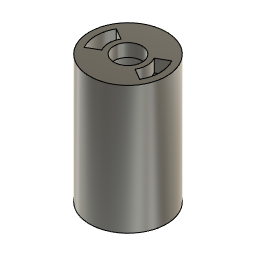
PDMSmould_holder (Autodesk Fusion 360 design; units mm, degrees)
Autodesk Fusion 360 part; units mm, degrees
sketch "Sketch1" plane through (0, 0, 0) normal (0, 0, 1) x (1, 0, 0)
  circle A0 centre (0, 0) radius 15
  dimension "d2" = 30
  constraint coincident A0.centre origin
  measures "d2" diameter of A0
extrude "Extrude1" add sketch "Sketch1" along normal blind 50
sketch "Sketch2" plane through (0, 0, 50) normal (0, 0, 1) x (-1, 0, 0)
  circle A0 centre (0, 0) radius 15
  circle A1 centre (0, 0) radius 12.5
  dimension "d5" = 25
  constraint concentric A0 A1
  measures "d5" diameter of A1
extrude "Extrude2" cut sketch "Sketch2" against normal blind 45 contours A1
sketch "Sketch4" plane through (0, 0, 50) normal (0, 0, 1) x (-1, 0, 0)
  circle A0 centre (0, 0) radius 12.5
  circle A1 centre (0, 0) radius 15
  circle A2 centre (0, 0) radius 15
  circle A3 centre (0, 0) radius 5.5
  dimension "d8" = 11
  constraint coincident A0.centre A1.centre
  measures "d8" diameter of A3
extrude "Extrude3" add sketch "Sketch4" against normal blind 5 contours A0
sketch "Sketch5" plane through (0, 0, 50) normal (0, 0, 1) x (-1, 0, 0)
  circle A0 centre (0, 0) radius 5.5
  circle A1 centre (0, 0) radius 15
  circle A2 centre (0, 0) radius 12.5
  circle A3 centre (0, 0) radius 7.5
  line L0 (0, 0) -> (12.5, 0) construction
  line L1 (0, 0) -> (-10.8253, 6.25)
  line L2 (0, 0) -> (12.5, 0) construction
  line L3 (0, 0) -> (-10.8253, -6.25)
  line L4 (0, 0) -> (12.5, 0) construction
  line L5 (0, 0) -> (10.8253, 6.25)
  line L6 (-10.8253, 6.25) -> (14.1746, 6.25) construction
  line L7 (0, 0) -> (10.8253, -6.25)
  line L8 (0, 0) -> (12.5, 0) construction
  dimension "d11" = 25
  dimension "d12" = 15
  dimension "d14" = 150
  dimension "d15" = 150
  dimension "d18" = 30
  constraint concentric A0 A2
  constraint concentric A2 A3
  constraint horizontal L0
  constraint coincident A0.centre A1.centre
  constraint horizontal L2
  constraint coincident A2 L1.end
  constraint horizontal L4
  constraint coincident A2 L3.end
  constraint coincident A2 L5.end
  constraint parallel L3 L5
  constraint horizontal L6
  constraint horizontal L8
  measures "d11" diameter of A2
  measures "d12" diameter of A3
  measures "d14" angle of L1 L2
  measures "d15" angle of L3 L4
  measures "d18" angle of L7 L8
extrude "Extrude4" cut sketch "Sketch5" against normal blind 5 contours A2 A3 L5 L7 | A2 A3 L1 L3
